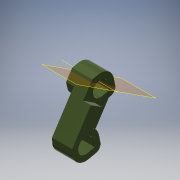
# Autodesk Inventor part: HbMiddle-RingCouplerLink01
Saved by Autodesk Inventor 2017 (Build 210142000, 142)
## iProperties
Created: 2015-02-23
Part Number: HbMiddle-RingCouplerLink01
Material: ナイロン 6/6
Document SubType Name: Modeling
Designer: Yamaura
Density: 1.13 g/cm^3
Appearance: 濃いオリーブ
Author: Yamaura
Autodesk Inventor part; units mm, degrees
ref_plane "YZ Plane" through (0, 0, 0) normal (1, 0, 0) x (0, 1, 0)
ref_plane "XZ Plane" through (0, 0, 0) normal (0, 1, 0) x (-1, 0, 0)
ref_plane "XY Plane" through (0, 0, 0) normal (0, 0, 1) x (1, 0, 0)
sketch "スケッチ1" plane through (0, 0, 0) normal (1, 0, 0) x (0, 1, 0)
  arc A0 (-2.5161, 1.6338) -> (2.5161, -1.6338) centre (0, 0) ccw
  circle A1 centre (5, 7.7) radius 1.7
  arc A2 (7.5161, 6.0662) -> (2.4839, 9.3338) centre (5, 7.7) ccw
  circle A3 centre (0, 0) radius 1.7
  line L0 (2.4839, 9.3338) -> (-2.5161, 1.6338)
  line L1 (7.5161, 6.0662) -> (2.5161, -1.6338)
  dimension "d1" = 3.4
  dimension "d2" = 6
  dimension "d3" = 3.4
  dimension "d4" = 5
  dimension "d5" = 7.7
  dimension "d8" = 3
  constraints: 4 centre point, 4 end point, 4 point on circle, 4 tangent, 3 coincident
  measures "d1" diameter of A1
  measures "d2" diameter of A2
  measures "d3" diameter of A3
  measures "d4" horizontal distance of A1.centre point (0, 0)
  measures "d5" vertical distance of A1.centre point (0, 0)
  measures "d8" radius of A0
extrude "押し出し1" add sketch "スケッチ1" against normal blind 6.2
sketch "スケッチ2" plane through (0, 0, 0) normal (1, 0, 0) x (0, 0, -1)
  circle A0 centre (0, 0) radius 1.7 projected
  circle A1 centre (-7.7, 5) radius 1.7 projected
  line L0 (-1.6338, -2.5161) -> (-9.3338, 2.4839) projected
  arc A2 (-1.6338, -2.5161) -> (1.6338, 2.5161) centre (0, 0) ccw projected
  line L1 (-6.0662, 7.5161) -> (1.6338, 2.5161) projected
  arc A3 (-6.0662, 7.5161) -> (-9.3338, 2.4839) centre (-7.7, 5) ccw projected
  circle A4 centre (0, 0) radius 3
  line L2 (-1.6338, -2.5161) -> (1.6338, 2.5161)
  dimension "d11" = 6
  constraints: 2 end point, 1 coincident, 1 midpoint, 1 perpendicular, 1 point on line, 3 other
extrude "押し出し2" cut sketch "スケッチ2" against normal blind 1.7 contours A4 L0 A3 L1
sketch "スケッチ3" plane through (-6.2, 0, 0) normal (-1, 0, 0) x (0, 0, 1)
  circle A0 centre (0, 0) radius 1.7 projected
  circle A1 centre (7.7, 5) radius 1.7 projected
  line L0 (1.6338, -2.5161) -> (9.3338, 2.4839) projected
  arc A2 (9.3338, 2.4839) -> (6.0662, 7.5161) centre (7.7, 5) ccw projected
  line L1 (6.0662, 7.5161) -> (-1.6338, 2.5161) projected
  arc A3 (-1.6338, 2.5161) -> (1.6338, -2.5161) centre (0, 0) ccw projected
  circle A4 centre (7.7, 5) radius 3
  line L2 (6.0662, 7.5161) -> (9.3338, 2.4839)
  line L3 (1.6338, -2.5161) -> (9.3338, 2.4839) projected
  dimension "d14" = 6
  constraints: 2 end point, 1 coincident, 1 midpoint, 1 perpendicular, 1 point on line, 3 other
extrude "押し出し3" cut sketch "スケッチ3" against normal blind 1.7 contours A4 L0 A3 L1
sketch "スケッチ5" plane through (-1.7, 0, 0) normal (1, 0, 0) x (0, 0, -1)
  arc A0 (-2.5161, 1.6338) -> (-1.6338, -2.5161) centre (0, 0) ccw
  line L0 (-1.6338, -2.5161) -> (-6.666, 0.7516)
  line L1 (-5.0322, 3.2676) -> (0, 0)
  line L2 (-6.666, 0.7516) -> (-5.0322, 3.2676)
  dimension "d18" = 6
  constraints: 6 end point, 2 point on circle, 1 centre point, 1 midpoint
  measures "d18" distance from line of L2 point (0, 0)
extrude "押し出し4" add sketch "スケッチ5" along normal up to surface (1.7 mm away)
move faces "移動1" translate (0, 0.3812, 0.5871) faces at (-1.1333, 2.4289, 5.5768)
sketch "スケッチ6" plane through (-4.5, 0, 0) normal (-1, 0, 0) x (0, 0, 1)
  arc A0 (6.0662, 7.5161) -> (9.3338, 2.4839) centre (7.7, 5) ccw projected
  line L0 (-1.6338, 2.5161) -> (6.0662, 7.5161) projected
  arc A1 (-1.6338, 2.5161) -> (1.6338, -2.5161) centre (0, 0) ccw projected
  line L1 (9.3338, 2.4839) -> (1.6338, -2.5161) projected
  circle A2 centre (0, 0) radius 1.7 projected
  line L2 (-2.3106, 3.5583) -> (-2.9344, 0.6239)
  line L3 (-2.3106, 3.5583) -> (0.6239, 2.9344)
  line L4 (0, 0) -> (-2.3106, 3.5583)
  arc A3 (-1.6338, 2.5161) -> (1.6338, -2.5161) centre (0, 0) ccw projected
  line L5 (9.3338, 2.4839) -> (1.6338, -2.5161) projected
  arc A4 (0.6239, 2.9344) -> (-2.9344, 0.6239) centre (0, 0) ccw
  dimension "d24" = 45
  constraints: 6 end point, 4 point on circle, 2 tangent, 1 centre point, 1 coincident, 1 perpendicular
  measures "d24" angle of L3 L4
extrude "押し出し5" add sketch "スケッチ6" against normal up to surface (4.5 mm away) contours L3 A4 L0 | L0 L4 L3 | A1 L2 L4
sketch "スケッチ7" plane through (-4.5, 0, 0) normal (-1, 0, 0) x (0, 0, 1)
  arc A0 (6.0662, 7.5161) -> (9.3338, 2.4839) centre (7.7, 5) ccw projected
  line L0 (-0.5916, 3.1928) -> (6.0662, 7.5161) projected
  arc A1 (-2.9344, 0.6239) -> (1.6338, -2.5161) centre (0, 0) ccw projected
  line L1 (9.3338, 2.4839) -> (1.6338, -2.5161) projected
  circle A2 centre (0, 0) radius 1.7 projected
  line L2 (-0.9258, 1.4258) -> (-1.3093, 2.0164)
  line L3 (-1.3093, 2.0164) -> (-1.6628, 0.3535)
  line L4 (-1.3093, 2.0164) -> (0.3535, 1.6628)
  circle A3 centre (0, 0) radius 1.7 projected
  line L5 (-0.5916, 3.1928) -> (-2.3106, 3.5583) projected
  line L6 (-2.3106, 3.5583) -> (-2.9344, 0.6239) projected
  dimension "d30" = 45
  constraints: 6 end point, 3 point on circle, 3 tangent, 1 perpendicular, 1 point on line
  measures "d30" angle of L4 L2
extrude "押し出し6" cut sketch "スケッチ7" against normal blind 10 contours A2 L2 L4 | L3 L2 A2
fillet "フィレット1" radius 1.3 1 edges at (-2.25, 3.5583, -2.3106)
sketch "スケッチ8" plane through (-6.2, 5, 7.7) normal (-1, 0, 0) x (0, 0, 1)
  circle A0 centre (0, 0) radius 3 projected
  circle A1 centre (0, 0) radius 1.7 projected
  line L0 (-1.6338, 2.5161) -> (-2.3106, 3.5583)
  line L1 (-2.3106, 3.5583) -> (-2.9344, 0.6239)
  circle A2 centre (0, 0) radius 3 projected
  line L2 (1.6338, -2.5161) -> (-6.0662, -7.5161) projected
  line L3 (-2.3106, 3.5583) -> (0.6239, 2.9344)
  point P0 (-7.7, -5)
  dimension "d35" = 45
  constraints: 6 end point, 3 point on circle, 2 tangent, 1 perpendicular, 1 point on line, 1 other
  measures "d35" angle of L0 L1
extrude "押し出し7" add sketch "スケッチ8" against normal up to surface (4.5 mm away) contours A0 L0 L3 | A0 L1 L0
fillet "フィレット2" radius 1.3 1 edges at (-3.95, 8.5583, 5.3894)
sketch "スケッチ9" plane through (-6.2, 0, 0) normal (-1, 0, 0) x (0, 0, 1)
  arc A0 (6.661, 8.2879) -> (5.1191, 7.2867) centre (6.3907, 7.0164) ccw projected
  line L0 (5.1191, 7.2867) -> (4.7656, 5.6239) projected
  arc A1 (4.7656, 5.6239) -> (8.3239, 7.9344) centre (7.7, 5) ccw projected
  line L1 (8.3239, 7.9344) -> (6.661, 8.2879) projected
  circle A2 centre (7.7, 5) radius 1.7 projected
  line L2 (6.7742, 6.4258) -> (6.3907, 7.0164)
  line L3 (9.3338, 2.4839) -> (1.6338, -2.5161) projected
  line L4 (6.3907, 7.0164) -> (8.0535, 6.6628)
  circle A3 centre (7.7, 5) radius 1.7 projected
  line L5 (6.3907, 7.0164) -> (6.0372, 5.3535)
  point P0 (0, 0)
  dimension "d40" = 45
  dimension "d41" = 45
  constraints: 6 end point, 3 point on circle, 2 tangent, 1 perpendicular, 1 point on line
  measures "d40" angle of L5 L2
  measures "d41" angle of L2 L4
extrude "押し出し8" cut sketch "スケッチ9" against normal blind 10 contours A2 L2 L4 | L5 L2 A2
sketch "スケッチ10" plane through (-6.2, 0, 0) normal (-1, 0, 0) x (0, 0, 1)
  line L0 (6.0372, 5.3535) -> (6.3907, 7.0164) projected
  line L1 (6.3907, 7.0164) -> (8.0535, 6.6628) projected
  arc A0 (6.0372, 5.3535) -> (8.0535, 6.6628) centre (7.7, 5) ccw projected
  arc A1 (6.661, 8.2879) -> (5.1191, 7.2867) centre (6.3907, 7.0164) ccw projected
  line L2 (5.1191, 7.2867) -> (4.7656, 5.6239) projected
  arc A2 (4.7656, 5.6239) -> (8.3239, 7.9344) centre (7.7, 5) ccw construction
  line L3 (8.3239, 7.9344) -> (6.661, 8.2879) projected
  line L4 (7.0761, 2.0656) -> (8.2916, 1.8072)
  arc A3 (4.7656, 5.6239) -> (8.3239, 7.9344) centre (7.7, 5) ccw projected
  line L5 (9.3338, 2.4839) -> (1.6338, -2.5161) projected
  line L6 (7.7, 5) -> (9.3338, 2.4839)
  arc A4 (7.0761, 2.0656) -> (9.3338, 2.4839) centre (7.7, 5) ccw
  line L7 (8.2916, 1.8072) -> (9.3338, 2.4839)
  point P0 (0, 0)
  point P1 (10.6344, 4.3761)
  dimension "d47" = 45
  constraints: 6 end point, 3 point on circle, 2 point on line, 2 symmetric about line, 2 tangent, 1 centre point, 1 coincident, 1 collinear, 1 perpendicular
  measures "d47" angle of L6 L4
extrude "押し出し10" add sketch "スケッチ10" against normal up to surface (4.5 mm away) contours L5 L4 A3
ref_plane "作業平面1" through (0, 5, 7.7) normal (0, 0.5446054, 0.8386924) x (-1, 0, 0)
mirror "ミラー1" about plane through (0, 5, 7.7) normal (0, 0.5446054, 0.8386924) of "押し出し10"
sketch "スケッチ11" plane through (0, 0, 0) normal (1, 0, 0) x (0, 0, -1)
  arc A0 (2.5809, 2.2867) -> (1.039, 3.2879) centre (1.3093, 2.0164) ccw projected
  line L0 (-0.6239, 2.9344) -> (1.039, 3.2879) projected
  arc A1 (-0.6239, 2.9344) -> (-2.5161, 1.6338) centre (0, 0) ccw projected
  line L1 (-5.6192, 3.6489) -> (-2.5161, 1.6338) projected
  line L2 (-7.2531, 1.1328) -> (-5.6192, 3.6489) projected
  line L3 (-1.6338, -2.5161) -> (-7.2531, 1.1328) projected
  arc A2 (-1.6338, -2.5161) -> (2.9344, 0.6239) centre (0, 0) ccw projected
  line L4 (2.5809, 2.2867) -> (2.9344, 0.6239) projected
  line L5 (-0.3535, 1.6628) -> (1.3093, 2.0164) projected
  line L6 (1.3093, 2.0164) -> (1.6628, 0.3535) projected
  arc A3 (-0.3535, 1.6628) -> (1.6628, 0.3535) centre (0, 0) ccw projected
  line L7 (0, 0) -> (-1.6338, -2.5161)
  line L8 (-1.6338, -2.5161) -> (-0.823, -3.0426)
  line L9 (-0.823, -3.0426) -> (0.1427, -2.9966)
  arc A4 (-1.6338, -2.5161) -> (0.1427, -2.9966) centre (0, 0) ccw
  constraints: 6 end point, 3 point on circle, 2 perpendicular, 1 centre point, 1 coincident, 1 point on line, 1 tangent
extrude "押し出し11" add sketch "スケッチ11" against normal up to surface (4.5 mm away) contours L9 L8 A2
scale "尺度1" factors (0.8836555, 0.8836555, 0.8836555) then translate (-0.5236, -0.0719, 0.5302) bodies 1
